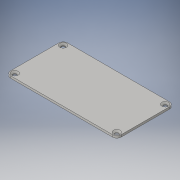
# Autodesk Inventor part: Frontplatte
Saved by Autodesk Inventor 2016 (Build 200138000, 138)
## iProperties
Created: 2018-04-27
Part Number: Frontplatte
Material: Generic
Document SubType Name: Modeling
Designer: Phil Erle
Density: 1 g/cm^3
Appearance: Default
Author: Phil Erle
Autodesk Inventor part; units mm, degrees
ref_plane "YZ Plane" through (0, 0, 0) normal (1, 0, 0) x (0, 1, 0)
ref_plane "XZ Plane" through (0, 0, 0) normal (0, 1, 0) x (-1, 0, 0)
ref_plane "XY Plane" through (0, 0, 0) normal (0, 0, 1) x (1, 0, 0)
sketch "Sketch1" plane through (0, 0, 0) normal (0, 0, 1) x (1, 0, 0)
  line L0 (-51.5, -26.5) -> (51.5, -26.5)
  line L1 (51.5, -26.5) -> (51.5, 26.5)
  line L2 (51.5, 26.5) -> (-51.5, 26.5)
  line L3 (-51.5, 26.5) -> (-51.5, -26.5)
  line L4 (-51.5, -26.5) -> (51.5, 26.5) construction
  line L5 (51.5, -26.5) -> (-51.5, 26.5) construction
  point P0 (0, 0)
  dimension "d0" = 103
  dimension "d1" = 53
  constraints: 12 end point, 2 midpoint, 2 parallel, 1 horizontal, 1 perpendicular
  measures "d0" distance of L1.end L2.end
  measures "d1" distance of L0.end L1.end
extrude "Extrusion1" add sketch "Sketch1" along normal blind 2
fillet "Fillet1" radius 4 4 edges at (-51.5, -26.5, 1) (-51.5, 26.5, 1) (51.5, -26.5, 1) (51.5, 26.5, 1)
sketch "Sketch2" plane through (0, 0, 2) normal (0, 0, 1) x (1, 0, 0)
  line L0 (-47.5, -22.5) -> (47.5, -22.5) construction
  line L1 (47.5, -22.5) -> (47.5, 22.5) construction
  line L2 (47.5, 22.5) -> (-47.5, 22.5) construction
  line L3 (-47.5, 22.5) -> (-47.5, -22.5) construction
  line L4 (-47.5, -22.5) -> (47.5, 22.5) construction
  line L5 (47.5, -22.5) -> (-47.5, 22.5) construction
  point P0 (0, 0)
  dimension "d5" = 95
  dimension "d6" = 45
  constraints: 12 end point, 4 coincident, 2 midpoint, 2 parallel, 1 horizontal, 1 perpendicular
  measures "d5" distance of L1.end L2.end
  measures "d6" distance of L2.end L0.start
hole "Hole1" at (-47.5, 22.5, 2) at (-47.5, -22.5, 2) at (47.5, -22.5, 2) at (47.5, 22.5, 2) direction (0, 0, -1) diameter 3.4 end through all countersink diameter 6.3 countersink angle 90 clearance for "Countersunk Flat Head Screw DIN EN ISO 2009" size "M3" standard "DIN"
body "Solid1"
